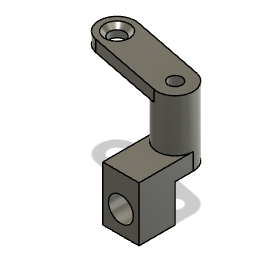
поворотный механизм тяга 1 (Autodesk Fusion 360 design; units mm, degrees)
Autodesk Fusion 360 part; units mm, degrees
note: some values were not read from the file. Set by a fixed rule: which sketch regions a step uses.
sketch "Sketch1" plane through (0, 0, 0) normal (0, 1, 0) x (1, 0, 0)
  line L0 (4, -4) -> (-4, -4)
  line L1 (-4, -4) -> (-4, 4)
  line L2 (-4, 4) -> (4, 4)
  line L3 (4, 4) -> (4, -4)
  line L4 (4, -4) -> (-4, 4) construction
  line L5 (-4, -4) -> (4, 4) construction
  dimension "d1" = 8
  dimension "d2" = 8
  constraint horizontal L0
  constraint perpendicular L0 L1
  constraint parallel L0 L2
  constraint parallel L1 L3
  constraint coincident L4 origin
  constraint coincident L5 origin
  measures "d1" distance of L1.end L2.end
  measures "d2" distance of L0.end L1.end
extrude "Extrude1" add sketch "Sketch1" along normal blind 8.3
sketch "Sketch2" plane through (0, 8.3, 0) normal (0, 1, 0) x (-1, 0, 0)
  line L0 (-4, -4) -> (4, -4)
  line L1 (4, -4) -> (4, 4)
  line L2 (4, 4) -> (-4, 4)
  line L3 (-4, 4) -> (-4, -4)
  line L4 (0, -4) -> (0, -12)
  circle A0 centre (0, -8) radius 4
  line L5 (4, -4) -> (4, -8)
  line L6 (-4, -4) -> (-4, -8)
  circle A1 centre (0, -8) radius 1.5
  dimension "d5" = 8
  dimension "d6" = 3
  constraint midpoint L0 L4.start
  constraint perpendicular L0 L4
  constraint midpoint L4 A0.centre
  constraint coincident L4.end A0
  constraint coincident L0.end L1.start
  constraint coincident A0 L5.end
  constraint tangent A0 L5
  constraint coincident L0.start L3.end
  constraint coincident A0 L6.end
  constraint tangent A0 L6
  constraint concentric A0 A1
  measures "d5" distance of L4.start L4.end
  measures "d6" diameter of A1
extrude "Extrude2" add sketch "Sketch2" along normal blind 3.75 contours L0 L1 L2 L3 | L0 A0 L6 | L4 A0 A1 | L0 A0 L5 | L4 A0 A1
sketch "Sketch3" plane through (0, 0, 4) normal (0, 0, 1) x (1, 0, 0)
  line L0 (-4, 0) -> (4, 0)
  line L1 (4, 0) -> (4, 12.05)
  line L2 (4, 12.05) -> (-4, 12.05)
  line L3 (-4, 12.05) -> (-4, 0)
  line L4 (0, 0) -> (0, 2.25)
  line L5 (0, 2.25) -> (0, 7.75)
  circle A0 centre (0, 5) radius 2.75
  dimension "d9" = 2.25
  dimension "d10" = 5.5
  constraint coincident L4.start origin
  constraint perpendicular L0 L4
  constraint parallel L4 L5
  constraint midpoint L5 A0.centre
  constraint coincident L5.end A0
  measures "d9" distance of L4.start L4.end
  measures "d10" distance of L4.end L5.end
extrude "Extrude3" cut sketch "Sketch3" against normal blind 20 contours L5 A0 | L5 A0
sketch "Sketch4" plane through (0, 12.05, 0) normal (0, 1, 0) x (-1, 0, 0)
  circle A0 centre (0, -8) radius 1.5
  line L0 (4, -8) -> (4, 4)
  line L1 (4, 4) -> (-4, 4)
  line L2 (-4, 4) -> (-4, -8)
  arc A1 (-4, -8) -> (4, -8) centre (0, -8) ccw
  circle A2 centre (0, -8) radius 4
  constraint concentric A0 A2
extrude "Extrude4" add sketch "Sketch4" along normal blind 11.5 contours A1 A2
sketch "Sketch5" plane through (0, 23.55, 0) normal (0, 1, 0) x (-1, 0, 0)
  circle A0 centre (0, -8) radius 1.5
  circle A1 centre (0, -8) radius 4
  line L0 (0, -8) -> (16, -11.1391)
  line L1 (0, -8) -> (16.305, -8) construction
  circle A2 centre (16, -11.1391) radius 4
  circle A3 centre (16, -11.1391) radius 1.75
  line L2 (8, -9.5695) -> (7.2299, -13.4947)
  line L3 (8, -9.5695) -> (8.7701, -5.6444)
  line L4 (7.2299, -13.4947) -> (15.2299, -15.0642)
  line L5 (8.7701, -5.6444) -> (16.7701, -7.2139)
  line L6 (8.7701, -5.6444) -> (0.7701, -4.0748)
  line L7 (7.2299, -13.4947) -> (-0.7701, -11.9252)
  dimension "d15" = 16.305
  dimension "d16" = 11.1
  dimension "d17" = 8
  dimension "d18" = 3.5
  dimension "d19" = 4
  dimension "d20" = 4
  constraint horizontal L1
  constraint coincident A0.centre A1.centre
  constraint coincident L0.end A2.centre
  constraint concentric A2 A3
  constraint midpoint L0 L2.start
  constraint perpendicular L0 L2
  constraint perpendicular L0 L3
  constraint coincident A2 L4.end
  constraint tangent A2 L4
  constraint coincident A2 L5.end
  constraint tangent A2 L5
  constraint coincident A1 L6.end
  constraint tangent A1 L6
  constraint coincident A1 L7.end
  constraint tangent A1 L7
  measures "d15" distance of A0.centre L0.end
  measures "d16" angle of L0 L1
  measures "d17" diameter of A2
  measures "d18" diameter of A3
  measures "d19" distance of L2.start L2.end
  measures "d20" distance of L2.start L3.end
extrude "Extrude5" add sketch "Sketch5" against normal blind 2.5 contours A1 L0 L3 L6 | A1 L0 L2 L7 | L0 A2 L3 L5 | L0 A2 L2 L4 | A2
chamfer "Chamfer1" distance 1 angle 45 1 edges at (-14.3684, 23.55, -10.5062)
